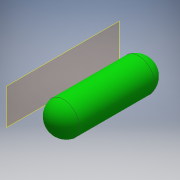
# Autodesk Inventor part: brazo
Saved by Autodesk Inventor 2016 (Build 200138000, 138)
## iProperties
Created: 2016-02-19
Part Number: brazo
Material: Genérico
Document SubType Name: Modeling
Designer: Usuario1
Density: 1 g/cm^3
Appearance: Valor por defecto
Author: Usuario1
Autodesk Inventor part; units mm, degrees
ref_plane "XZ Plane" through (0, 0, 0) normal (0, 1, 0) x (-1, 0, 0)
ref_plane "XY Plane" through (0, 0, 0) normal (0, 0, 1) x (1, 0, 0)
sketch "Boceto1" plane through (0, 0, 0) normal (0, 0, 1) x (1, 0, 0)
  line L0 (-1.2847, 0.7744) -> (-1.2847, 6.7094)
  line L1 (-0.9847, 0.8029) -> (-0.9847, 6.6809)
  arc A0 (-1.2847, 0.7744) -> (0, -0.3) centre (0, 1.0052) ccw
  arc A1 (-0.9847, 0.8029) -> (0, 0) centre (0, 1.0052) ccw
  arc A2 (0, 7.7838) -> (-1.2847, 6.7094) centre (0, 6.4786) ccw
  arc A3 (0, 7.4838) -> (-0.9847, 6.6809) centre (0, 6.4786) ccw
  line L2 (0, 0) -> (0, -0.3)
  line L3 (0, 7.4838) -> (0, 7.7838)
  line L4 (0, 7.4838) -> (0, 4.9838)
  line L5 (0, 4.9838) -> (-0.9847, 4.9838)
  line L6 (-0.9847, 6.6809) -> (-0.9847, 4.9838)
  point P0 (0, 0)
  dimension "d2" = 2.5
  constraints: 14 end point, 8 point on circle, 4 centre point, 2 perpendicular, 1 point on line, 1 vertical
  measures "d2" distance of L3.start L4.end
revolve "Revolución1" add sketch "Boceto1" angle 360 about axis through (0, 7.4838, 0) along (0, 1, 0)
ref_plane "Plano de trabajo1" through (-3, 0, 0) normal (1, 0, 0) x (0, 1, 0)
sketch "Boceto2" plane through (-3, 0, 0) normal (1, 0, 0) x (0, 1, 0)
  line L0 (0.7744, -1.2847) -> (0.7744, 1.2847) projected
  arc A0 (0.7744, 1.2847) -> (0.7744, -1.2847) centre (1.0052, 0) ccw projected
  line L1 (0.7744, 1.2847) -> (6.7094, 1.2847)
  line L2 (0.8029, 0.9847) -> (6.6809, 0.9847)
  arc A1 (0.7744, 1.2847) -> (-0.3, 0) centre (1.0052, 0) ccw
  arc A2 (0.8029, 0.9847) -> (0, 0) centre (1.0052, 0) ccw
  arc A3 (7.7838, 0) -> (6.7094, 1.2847) centre (6.4786, 0) ccw
  arc A4 (7.4838, 0) -> (6.6809, 0.9847) centre (6.4786, 0) ccw
  line L3 (6.4094, 0.4) -> (6.4094, -0.4)
  line L4 (5.6094, -0.4) -> (5.6094, 0.4)
  line L5 (0, 0) -> (-0.3, 0)
  line L6 (7.4838, 0) -> (7.7838, 0)
  line L7 (6.4094, 0.4) -> (5.6094, 0.4)
  line L8 (6.4094, -0.4) -> (5.6094, -0.4)
  point P0 (0, 0)
  constraints: 16 end point, 8 point on circle, 4 centre point
extrude "Extrusión1" cut sketch "Boceto2" along normal blind 3 contours L3 L8 L4 L7
